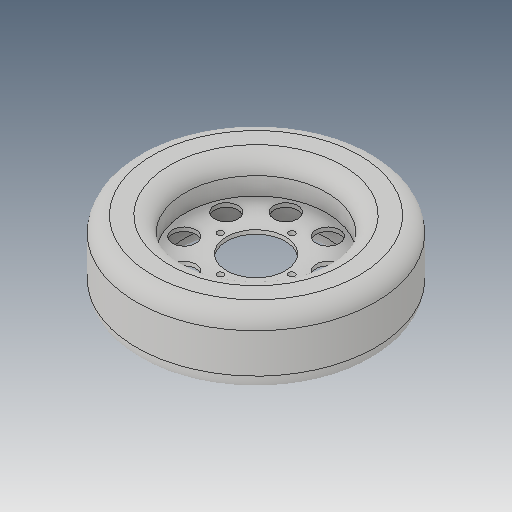
# Autodesk Inventor part: 車輪
Saved by Autodesk Inventor 2020.3 (Build 243373000, 373)
## iProperties
Part Number: 車輪
Material: 一般
Document SubType Name: Modeling
Designer: highs
Density: 1 g/cm^3
Appearance: 既定
Description: https://store.shopping.yahoo.co.jp/redmotoparts/ca085.html
Stock Number: モンキー・ゴリラ用　８インチ　アルミホイール・タイヤセット
Author: highs
Revision Number: ホイール2.5J  タイヤ90/65-8　組付けオプション申し込み
Autodesk Inventor part; units mm, degrees
ref_plane "YZ Plane" through (0, 0, 0) normal (1, 0, 0) x (0, 1, 0)
ref_plane "XZ Plane" through (0, 0, 0) normal (0, 1, 0) x (-1, 0, 0)
ref_plane "XY Plane" through (0, 0, 0) normal (0, 0, 1) x (1, 0, 0)
sketch "スケッチ1" plane through (0, 0, 0) normal (0, 0, 1) x (1, 0, 0)
  line L0 (0, 0) -> (90, 0)
  line L1 (90, 0) -> (90, -42.5)
  line L2 (90, -42.5) -> (152, -42.5)
  line L3 (152, -42.5) -> (152, 47.5)
  line L4 (152, 47.5) -> (90, 47.5)
  line L5 (90, 47.5) -> (90, 5)
  line L6 (90, 5) -> (0, 5)
  line L7 (0, 5) -> (0, 0)
  line L8 (0, 2.5) -> (152, 2.5) construction
  dimension "d0" = 5
  dimension "d1" = 152
  dimension "d2" = 90
  dimension "d3" = 90
  constraints: 18 end point, 6 perpendicular, 2 horizontal, 2 midpoint, 2 point on line
  measures "d0" distance between parallel lines of L6 L0
  measures "d1" distance between parallel lines of L7 L3
  measures "d2" distance of L5.end L6.end
  measures "d3" distance of L2.end L3.end
revolve "回転1" add sketch "スケッチ1" angle 360 about axis through (0, 5, 0) along (0, -1, 0)
sketch "スケッチ2" plane through (0, 5, 0) normal (0, 1, 0) x (1, 0, 0)
  circle A0 centre (0, 0) radius 37.5
  circle A1 centre (0, 45.5) radius 4
  line L0 (0, 0) -> (0, 45.5) construction
  circle A2 centre (-45.5, 0) radius 4
  circle A3 centre (0, -45.5) radius 4
  circle A4 centre (45.5, 0) radius 4
  line L1 (0, 0) -> (26.7878, 64.6716) construction
  circle A5 centre (26.7878, 64.6716) radius 15
  circle A6 centre (0, 0) radius 70 construction
  circle A7 centre (-26.7878, 64.6716) radius 15
  circle A8 centre (-64.6716, 26.7878) radius 15
  circle A9 centre (-64.6716, -26.7878) radius 15
  circle A10 centre (-26.7878, -64.6716) radius 15
  circle A11 centre (26.7878, -64.6716) radius 15
  circle A12 centre (64.6716, -26.7878) radius 15
  circle A13 centre (64.6716, 26.7878) radius 15
  dimension "d18" = 140
  dimension "d6" = 45.5
  dimension "d7" = 8
  dimension "d8" = 75
  dimension "d11" = 360
  dimension "d16" = 22.5
  dimension "d17" = 30
  dimension "d21" = 360
  constraints: 13 centre point, 4 end point, 3 coincident, 1 vertical, 29 other
  measures "d6" distance of L0.start L0.end
  measures "d7" diameter of A1
  measures "d8" diameter of A0
  measures "d16" angle of L0 L1
  measures "d17" diameter of A5
extrude "押し出し1" cut sketch "スケッチ2" against normal up to next
fillet "フィレット1" radius 20 4 edges at (-152, 47.5, 0) (-152, -42.5, 0) (-90, 47.5, 0) (-90, -42.5, 0)
